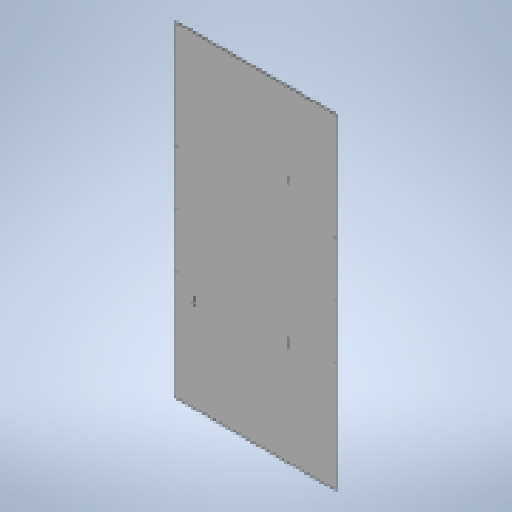
# Autodesk Inventor part: GBK 3328 shield 8
Saved by Autodesk Inventor 2026 (Build 300175000, 175)
## iProperties
Created: 2026-04-17
Part Number: GBK 3328 shield 8
Material: Steel
Document SubType Name: Sheet Metal
Designer: pokla
Stock Number: 3328
Mass: 69243.3 g
Surface Area: 44341.6 cm^2
Volume: 8820.8 cm^3
Density: 7.85 g/cm^3
Flat Pattern Width: 148 cm
Flat Pattern Length: 298 cm
Flat Pattern Area: 44104 cm^2
Sheet Metal Rule: По умолчанию_мм
Sheet Metal Width: 1480,000 мм
Sheet Metal Length: 2980,000 мм
Sheet Metal Area: 4410400,000 мм^2
Appearance: Default
Author: admin
Autodesk Inventor part; units mm, degrees
ref_plane "YZ Plane" through (0, 0, 0) normal (1, 0, 0) x (0, 1, 0)
ref_plane "XZ Plane" through (0, 0, 0) normal (0, 1, 0) x (-1, 0, 0)
ref_plane "XY Plane" through (0, 0, 0) normal (0, 0, 1) x (1, 0, 0)
sketch "Sketch1" plane through (0, 0, 0) normal (0, 0, 1) x (1, 0, 0)
  line L0 (740, -1490) -> (-740, -1490)
  line L1 (-740, -1490) -> (-740, 1490)
  line L2 (-740, 1490) -> (740, 1490)
  line L3 (740, 1490) -> (740, -1490)
  line L4 (740, -1490) -> (-740, 1490) construction
  line L5 (-740, -1490) -> (740, 1490) construction
  point P0 (0, 0)
  dimension "d0" = 1480
  dimension "d1" = 2980
  measures "d0" distance of L1.end L2.end
  measures "d1" distance of L0.end L1.end
extrude "Plate1" add sketch "Sketch1" along normal blind 4
sketch "Эскиз3" plane through (0, 0, 0) normal (0, 0, -1) x (-1, 0, 0)
  line L0 (567.5874, -1279.3136) -> (567.5874, -1777.4498) construction
  line L1 (567.5874, -1777.4498) -> (527.9602, -1777.4498) construction
  line L2 (527.9602, -1777.4498) -> (527.9602, -1279.3136) construction
  line L3 (527.9602, -1279.3136) -> (567.5874, -1279.3136) construction
  line L4 (209.363, -1239.5) -> (209.363, -1336.5) projected
  line L5 (209.363, -1336.5) -> (205.363, -1336.5) projected
  line L6 (-290.5101, -1239.5) -> (-290.5101, -1336.5) projected
  line L7 (-290.5101, -1336.5) -> (-294.5101, -1336.5) projected
  line L8 (209.363, 1458.5) -> (209.363, 1518.5) projected
  line L9 (209.363, 1458.5) -> (205.363, 1458.5) projected
  line L10 (-290.5101, 1458.5) -> (-290.5101, 1518.5) projected
  line L11 (-290.5101, 1458.5) -> (-294.5101, 1458.5) projected
  line L12 (-740, 1247.335) -> (-710, 1247.335) projected
  line L13 (-710, 1247.335) -> (-710, 1251.335) projected
  line L14 (-740, 750.668) -> (-710, 750.668) projected
  line L15 (-710, 750.668) -> (-710, 754.668) projected
  line L16 (-740, 254.001) -> (-710, 254.001) projected
  line L17 (-710, 254.001) -> (-710, 258.001) projected
  line L18 (-740, -242.666) -> (-710, -242.666) projected
  line L19 (-710, -242.666) -> (-710, -238.666) projected
  line L20 (-740, -739.333) -> (-710, -739.333) projected
  line L21 (-710, -739.333) -> (-710, -735.333) projected
  line L22 (-740, -1236) -> (-710, -1236) projected
  line L23 (-710, -1236) -> (-710, -1232) projected
  line L24 (739.6246, -1236) -> (739.6246, -1232) projected
  line L25 (739.6246, -739.333) -> (739.6246, -735.333) projected
  line L26 (739.6246, -242.666) -> (739.6246, -238.666) projected
  line L27 (739.6246, 254.001) -> (739.6246, 258.001) projected
  line L28 (739.6246, 750.668) -> (739.6246, 754.668) projected
  line L29 (739.6246, 1247.335) -> (739.6246, 1251.335) projected
  line L30 (739.6246, -1236) -> (709.6246, -1236)
  line L31 (739.6246, -739.333) -> (709.6246, -739.333)
  line L32 (739.6246, -242.666) -> (709.6246, -242.666)
  line L33 (739.6246, 254.001) -> (709.6246, 254.001)
  line L34 (739.6246, 750.668) -> (709.6246, 750.668)
  line L35 (739.6246, 1247.335) -> (709.6246, 1247.335)
  point P0 (0, 0)
  dimension "d6" = 30
  dimension "d7" = 30
  dimension "d8" = 30
  dimension "d9" = 30
  dimension "d10" = 30
  dimension "d11" = 30
  constraints: 12 end point, 6 horizontal, 2 other
  measures "d6" distance of L24.start L30.end
  measures "d7" distance of L31.start L31.end
  measures "d8" distance of L32.start L32.end
  measures "d9" distance of L33.start L33.end
  measures "d10" distance of L34.start L34.end
  measures "d11" distance of L35.start L35.end
mark "Маркировка2"
equation "\"d0\" = Лист_ширина"
equation "\"d2\" = Thickness"
equation "\"BendRadius\" = Thickness"
equation "\"BendReliefWidth\" = Thickness"
equation "\"BendReliefDepth\" = 0.5 * Thickness"
equation "\"CornerReliefSize\" = 4 * Thickness"
equation "\"MinimumRemnant\" = 2 * Thickness"
equation "\"TransitionRadius\" = BendRadius"
equation "\"JacobiRadiusSize\" = BendRadius"
equation "\"GapSize\" = Thickness"
equation "\"Лист_ширина\" = 1480"
equation "\"Thickness\" = 4"
body "Solid1"
